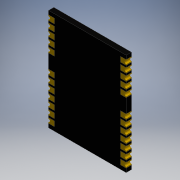
# Autodesk Inventor part: NEO-7
Saved by Autodesk Inventor 2016 (Build 200138000, 138)
## iProperties
Created: 2016-07-18
Part Number: NEO-7
Material: Generic
Document SubType Name: Modeling
Designer: Jonathan
Density: 1 g/cm^3
Appearance: Default
Author: Jonathan
Autodesk Inventor part; units mm, degrees
ref_plane "YZ Plane" through (0, 0, 0) normal (1, 0, 0) x (0, 1, 0)
ref_plane "XZ Plane" through (0, 0, 0) normal (0, 1, 0) x (-1, 0, 0)
ref_plane "XY Plane" through (0, 0, 0) normal (0, 0, 1) x (1, 0, 0)
sketch "Sketch1" plane through (0, 0, 0) normal (0, 1, 0) x (-1, 0, 0)
  line L0 (6.1, 8) -> (-6.1, 8)
  line L1 (-6.1, 8) -> (-6.1, -8)
  line L2 (-6.1, -8) -> (6.1, -8)
  line L3 (6.1, -8) -> (6.1, 8)
  point P0 (0, 0)
  point P1 (6.1, 0)
  point P2 (0, -8)
  dimension "d0" = 12.2
  dimension "d1" = 16
  constraints: 8 end point, 2 midpoint, 2 parallel, 1 horizontal, 1 horizontal alignment, 1 perpendicular, 1 vertical alignment
  measures "d0" distance of L0.start L0.end
  measures "d1" distance of L2.end L0.start
extrude "Extrusion1" add sketch "Sketch1" along normal blind 0.82
sketch "Sketch2" plane through (0, 0.82, 0) normal (0, 1, 0) x (1, 0, 0)
  line L0 (-6.1, -7.4) -> (-5.2, -7.4)
  line L1 (-5.2, -7.4) -> (-5.2, -6.6)
  line L2 (-5.2, -6.6) -> (-6.1, -6.6)
  line L3 (-6.1, -6.6) -> (-6.1, -7.4)
  line L4 (-6.1, 8) -> (-6.1, -8) projected
  line L5 (-6.1, -6.3) -> (-5.2, -6.3)
  line L6 (-5.2, -6.3) -> (-5.2, -5.5)
  line L7 (-5.2, -5.5) -> (-6.1, -5.5)
  line L8 (-6.1, -5.5) -> (-6.1, -6.3)
  line L9 (-6.1, -5.2) -> (-5.2, -5.2)
  line L10 (-5.2, -5.2) -> (-5.2, -4.4)
  line L11 (-5.2, -4.4) -> (-6.1, -4.4)
  line L12 (-6.1, -4.4) -> (-6.1, -5.2)
  line L13 (-6.1, -4.1) -> (-5.2, -4.1)
  line L14 (-5.2, -4.1) -> (-5.2, -3.3)
  line L15 (-5.2, -3.3) -> (-6.1, -3.3)
  line L16 (-6.1, -3.3) -> (-6.1, -4.1)
  line L17 (-6.1, -3) -> (-5.2, -3)
  line L18 (-5.2, -3) -> (-5.2, -2.2)
  line L19 (-5.2, -2.2) -> (-6.1, -2.2)
  line L20 (-6.1, -2.2) -> (-6.1, -3)
  line L21 (-6.1, -8) -> (6.1, -8) projected
  line L22 (-6.1, 2.2) -> (-5.2, 2.2)
  line L23 (-5.2, 2.2) -> (-5.2, 3)
  line L24 (-5.2, 3) -> (-6.1, 3)
  line L25 (-6.1, 3) -> (-6.1, 2.2)
  line L26 (-6.1, 3.3) -> (-5.2, 3.3)
  line L27 (-5.2, 3.3) -> (-5.2, 4.1)
  line L28 (-5.2, 4.1) -> (-6.1, 4.1)
  line L29 (-6.1, 4.1) -> (-6.1, 3.3)
  line L30 (-6.1, 4.4) -> (-5.2, 4.4)
  line L31 (-5.2, 4.4) -> (-5.2, 5.2)
  line L32 (-5.2, 5.2) -> (-6.1, 5.2)
  line L33 (-6.1, 5.2) -> (-6.1, 4.4)
  line L34 (-6.1, 5.5) -> (-5.2, 5.5)
  line L35 (-5.2, 5.5) -> (-5.2, 6.3)
  line L36 (-5.2, 6.3) -> (-6.1, 6.3)
  line L37 (-6.1, 6.3) -> (-6.1, 5.5)
  line L38 (-6.1, 6.6) -> (-5.2, 6.6)
  line L39 (-5.2, 6.6) -> (-5.2, 7.4)
  line L40 (-5.2, 7.4) -> (-6.1, 7.4)
  line L41 (-6.1, 7.4) -> (-6.1, 6.6)
  line L42 (6.1, 8) -> (-6.1, 8) projected
  line L43 (-6.1, 1.9) -> (-5.2, 1.9)
  line L44 (-5.2, 1.9) -> (-5.2, 1.1)
  line L45 (-5.2, 1.1) -> (-6.1, 1.1)
  line L46 (-6.1, 1.1) -> (-6.1, 1.9)
  line L47 (-6.1, 0.8) -> (-5.2, 0.8)
  line L48 (-5.2, 0.8) -> (-5.2, 0)
  line L49 (-5.2, 0) -> (-6.1, 0)
  line L50 (-6.1, 0) -> (-6.1, 0.8)
  point P0 (0, 0)
  point P1 (-5.2, -7)
  point P2 (-5.2, -5.9)
  point P3 (-5.2, -4.8)
  point P4 (-5.2, -3.7)
  point P5 (-5.2, -2.6)
  point P6 (-5.2, 2.6)
  point P7 (-5.2, 3.7)
  point P8 (-5.2, 4.8)
  point P9 (-5.2, 5.9)
  point P10 (-5.2, 7)
  point P11 (-5.2, 1.5)
  point P12 (-5.2, 0.4)
  dimension "d4" = 0.9
  dimension "d5" = 0.8
  dimension "d6" = 1.1
  dimension "d7" = 1.1
  dimension "d8" = 1.1
  dimension "d9" = 1.1
  dimension "d10" = 1
  dimension "d11" = 0.9
  dimension "d12" = 0.8
  dimension "d13" = 1.1
  dimension "d14" = 1.1
  dimension "d15" = 1.1
  dimension "d16" = 1.1
  dimension "d17" = 1
  dimension "d18" = 0.8
  dimension "d19" = 0.8
  dimension "d21" = 1.1
  dimension "d22" = 1.1
  constraints: 96 end point, 24 parallel, 15 collinear, 15 point on line, 12 horizontal, 12 midpoint, 12 perpendicular
  measures "d4" distance of L0.start L0.end
  measures "d5" distance of L0.end L1.end
  measures "d6" distance of point (-5.2, -5.9) point (-5.2, -7)
  measures "d7" distance of point (-5.2, -4.8) point (-5.2, -5.9)
  measures "d8" distance of point (-5.2, -3.7) point (-5.2, -4.8)
  measures "d9" distance of point (-5.2, -2.6) point (-5.2, -3.7)
  measures "d10" distance from line of L21 point (-5.2, -7)
  measures "d11" distance of L22.start L22.end
  measures "d12" distance of L22.end L23.end
  measures "d13" distance of point (-5.2, 3.7) point (-5.2, 2.6)
  measures "d14" distance of point (-5.2, 4.8) point (-5.2, 3.7)
  measures "d15" distance of point (-5.2, 5.9) point (-5.2, 4.8)
  measures "d16" distance of point (-5.2, 7) point (-5.2, 5.9)
  measures "d17" distance from line of L42 point (-5.2, 7)
  measures "d18" distance of L43.end L44.end
  measures "d19" distance of L47.end L48.end
  measures "d21" distance of point (-5.2, 1.5) point (-5.2, 2.6)
  measures "d22" distance of point (-5.2, 0.4) point (-5.2, 1.5)
extrude "Extrusion2" cut sketch "Sketch2" against normal blind 0.82
extrude "Extrusion3" add sketch "Sketch2" against normal blind 0.82 separate body
sketch "Sketch3" plane through (0, 0.82, 0) normal (0, 1, 0) x (1, 0, 0)
  line L0 (-6.1, -7.4) -> (-6.1, -6.6) projected
  circle A0 centre (-6.1, -7) radius 0.25
  line L1 (-6.1, -5.5) -> (-6.1, -6.3) projected
  circle A1 centre (-6.1, -5.9) radius 0.25
  line L2 (-6.1, -5.2) -> (-6.1, -4.4) projected
  circle A2 centre (-6.1, -4.8) radius 0.25
  line L3 (-6.1, -4.1) -> (-6.1, -3.3) projected
  circle A3 centre (-6.1, -3.7) radius 0.25
  line L4 (-6.1, -3) -> (-6.1, -2.2) projected
  circle A4 centre (-6.1, -2.6) radius 0.25
  line L5 (-6.1, 0.8) -> (-6.1, 0) projected
  circle A5 centre (-6.1, 0.4) radius 0.25
  line L6 (-6.1, 1.1) -> (-6.1, 1.9) projected
  circle A6 centre (-6.1, 1.5) radius 0.25
  line L7 (-6.1, 2.2) -> (-6.1, 3) projected
  circle A7 centre (-6.1, 2.6) radius 0.25
  circle A8 centre (-6.1, 3.7) radius 0.25
  line L8 (-6.1, 4.4) -> (-6.1, 5.2) projected
  circle A9 centre (-6.1, 4.8) radius 0.25
  line L9 (-6.1, 5.5) -> (-6.1, 6.3) projected
  circle A10 centre (-6.1, 5.9) radius 0.25
  line L10 (-6.1, 6.6) -> (-6.1, 7.4) projected
  circle A11 centre (-6.1, 7) radius 0.25
  line L11 (-6.1, 3.3) -> (-6.1, 4.1) projected
  point P0 (0, 0)
  dimension "d28" = 0.5
  constraints: 12 centre point, 12 midpoint, 11 equal radius, 1 coincident
  measures "d28" diameter of A0
extrude "Extrusion4" cut sketch "Sketch3" against normal blind 0.82 bodies 2
mirror "Mirror3" about plane through (0, 0, 0) normal (1, 0, 0) of "Extrusion2" bodies 1
mirror "Mirror4" about plane through (0, 0, 0) normal (1, 0, 0) of "Extrusion3", "Extrusion4" bodies 2
body "Solid1"
body "Solid2"
